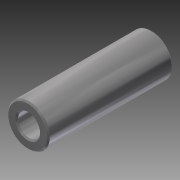
# Autodesk Inventor part: BearingLinearLMUW8
Saved by Autodesk Inventor 2015 SP1 (Build 190203100, 203)
## iProperties
Category: Hardware
Created: 2014-08-25
Part Number: BearingLinearLMUW8
Material: Steel, Alloy
Document SubType Name: Modeling
Designer: t_clevj
Density: 7.73 g/cm^3
Appearance: Semi-Polished
Mass: 43.8457 g
Surface Area: 34.6212 cm^2
Volume: 5.67215 cm^3
Vendor: Misumi
Catalog Web Link: http://us.misumi-ec.com/vona2/detail/110300026540/
Author: Jack
Title: Bearing Linear LMU8
Autodesk Inventor part; units mm, degrees
ref_plane "YZ Plane" through (0, 0, 0) normal (1, 0, 0) x (0, 1, 0)
ref_plane "XZ Plane" through (0, 0, 0) normal (0, 1, 0) x (-1, 0, 0)
ref_plane "XY Plane" through (0, 0, 0) normal (0, 0, 1) x (1, 0, 0)
sketch "Sketch1" plane through (0, 0, 0) normal (0, 1, 0) x (-1, 0, 0)
  circle A0 centre (0, 0) radius 4
  circle A1 centre (0, 0) radius 7.5
  dimension "d0" = 8
  dimension "d1" = 15
  constraints: 2 centre point, 2 coincident
  measures "d0" diameter of A0
  measures "d1" diameter of A1
extrude "Extrusion1" add sketch "Sketch1" along normal blind 45
chamfer "Chamfer1" distance 0.5 angle 45 4 edges at (7.5, 45, 0) (4, 45, 0) (7.5, 0, 0) (4, 0, 0)
body "Solid1"
